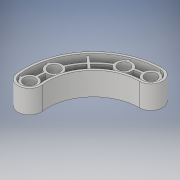
# Autodesk Inventor part: Curved_beam_6h-03
Saved by Autodesk Inventor 2019.3 (Build 233278000, 278)
## iProperties
Created: 2019-01-29
Part Number: Curved_beam_6h-03
Material: Generic
Document SubType Name: Modeling
Designer: Varga Daniel
Density: 1 g/cm^3
Appearance: Default
Inner_diameter: 40,000 mm
End_hole_dist: 37,500 mm
Author: Varga Daniel
Autodesk Inventor part; units mm, degrees
ref_plane "YZ Plane" through (0, 0, 0) normal (1, 0, 0) x (0, 1, 0)
ref_plane "XZ Plane" through (0, 0, 0) normal (0, 1, 0) x (-1, 0, 0)
ref_plane "XY Plane" through (0, 0, 0) normal (0, 0, 1) x (1, 0, 0)
derived "Base_part.ipt"
sketch "Sketch2" plane through (0, 0, 0) normal (0, 1, 0) x (-1, 0, 0)
  arc A0 (0, -20) -> (19.8431, 2.5) centre (0, 0) ccw
  arc A1 (0, -25) -> (24.8039, 3.125) centre (0, 0) ccw construction
  arc A2 (0, -30) -> (29.7647, 3.75) centre (0, 0) ccw
  line L0 (0, -20) -> (0, -30) construction
  line L1 (19.8431, 2.5) -> (29.7647, 3.75) construction
  arc A3 (0, -21) -> (20.8353, 2.625) centre (0, 0) ccw
  arc A4 (0, -29) -> (28.7725, 3.625) centre (0, 0) ccw
  circle A5 centre (0, -25) radius 3.5
  circle A6 centre (9.798, -23) radius 3.5
  arc A7 (0, -20) -> (0, -30) centre (0, -25) ccw
  arc A8 (0, -21) -> (0, -29) centre (0, -25) ccw
  arc A9 (29.7647, 3.75) -> (19.8431, 2.5) centre (24.8039, 3.125) ccw
  arc A10 (28.7725, 3.625) -> (20.8353, 2.625) centre (24.8039, 3.125) ccw
  circle A11 centre (24.8039, 3.125) radius 3.5
  circle A12 centre (24.0443, -6.8461) radius 3.5
  line L2 (0, 0) -> (22.5, -19.8431) construction
  arc A13 (24.6256, 6.6205) -> (24.488, 7.1125) centre (0, 0) ccw
  arc A14 (23.6421, 6.4265) -> (23.5058, 6.9085) centre (0, 0) ccw
  arc A15 (24.2694, -3.3534) -> (24.4973, -0.3615) centre (0, 0) ccw
  arc A16 (25.2502, -3.5604) -> (25.4982, -0.3055) centre (0, 0) ccw
  arc A17 (12.6551, -20.9785) -> (22.3958, -9.9336) centre (0, 0) ccw
  arc A18 (13.111, -21.8713) -> (23.3386, -10.2742) centre (0, 0) ccw
  arc A19 (-3.9161, -24.185) -> (-3.4209, -24.26) centre (0, 0) ccw
  arc A20 (3.4209, -24.26) -> (6.3607, -23.6599) centre (0, 0) ccw
  arc A21 (-3.9957, -25.185) -> (-3.4903, -25.26) centre (0, 0) ccw
  arc A22 (3.4903, -25.26) -> (6.6888, -24.6071) centre (0, 0) ccw
  line L3 (0, -25) -> (0, 0) construction
  line L4 (9.798, -23) -> (0, 0) construction
  line L5 (24.0443, -6.8461) -> (0, 0) construction
  line L6 (24.8039, 3.125) -> (0, 0) construction
  line L7 (7.768, -19.5105) -> (7.9803, -20.009)
  line L8 (10.6956, -26.3829) -> (10.9039, -26.872)
  line L9 (8.688, -19.1186) -> (8.9003, -19.6171)
  line L10 (11.6156, -25.991) -> (11.8239, -26.4801)
  line L11 (0.5, -20.994) -> (0.5, -21.5359)
  line L12 (0.5, -28.4641) -> (0.5, -28.9957)
  line L13 (-0.5, -28.9686) -> (-0.5, -28.4641)
  line L14 (-0.5, -21.5359) -> (-0.5, -21.0314)
  circle A23 centre (0, -25) radius 2.5
  circle A24 centre (9.798, -23) radius 2.5
  circle A25 centre (24.0443, -6.8461) radius 2.5
  circle A26 centre (24.8039, 3.125) radius 2.5
  line L15 (20.0546, -6.23) -> (20.5757, -6.3784)
  line L16 (27.2391, -8.2756) -> (27.7504, -8.4212)
  line L17 (20.3285, -5.2682) -> (20.8496, -5.4166)
  line L18 (27.513, -7.3138) -> (28.0242, -7.4594)
  line L19 (28.6789, 4.1172) -> (28.1784, 4.0541)
  line L20 (21.3045, 3.1881) -> (20.8039, 3.125)
  line L21 (20.8919, 2.1282) -> (21.4295, 2.1959)
  line L22 (28.3034, 3.0619) -> (28.8308, 3.1284)
  circle A27 centre (5, 5) radius 2.5 construction
  circle A28 centre (5, 5) radius 3.5 construction
  line L23 (15.4148, -14.2613) -> (18.0405, -16.5769)
  line L24 (18.7019, -15.8269) -> (16.0763, -13.5113)
  line L25 (18.7906, -17.2384) -> (21.416, -19.5538)
  line L26 (22.0775, -18.8038) -> (19.452, -16.4884)
  dimension "d84" = 7
  dimension "d85" = 7
  dimension "d86" = 7
  dimension "d87" = 7
  dimension "d0" = 20
  dimension "d5" = 1
  dimension "d14" = 10
  dimension "d15" = 4
  dimension "d21" = 10
  dimension "d34" = 1
  dimension "d35" = 0.5
  dimension "d37" = 1
  dimension "d38" = 1
  dimension "d45" = 5
  dimension "d51" = 1
  dimension "d53" = 1
  dimension "d77" = 4
  dimension "d78" = 4
  dimension "d79" = 5
  dimension "d80" = 7
  dimension "d81" = 5
  dimension "d82" = 5
  dimension "d83" = 5
  dimension "d88" = 1
  dimension "d89" = 37.5
  constraints: 54 end point, 51 point on circle, 21 centre point, 17 parallel, 12 coincident, 10 collinear, 8 concentric, 7 point on line, 3 midpoint, 2 vertical, 1 tangent, 74 other
  measures "d0" radius of A0
  measures "d14" distance of A1.start L4.start
  measures "d15" radius of A8
  measures "d21" distance of A9.centre L5.start
  measures "d34" radial gap between concentric circles of A20 A22
  measures "d35" radial gap between concentric circles of A1 A22
  measures "d37" distance between parallel lines of L14 L11
  measures "d38" distance between parallel lines of L7 L9
  measures "d45" diameter of A25
  measures "d51" distance between parallel lines of L17 L15
  measures "d53" distance between parallel lines of L20 L21
  measures "d79" diameter of A27
  measures "d80" diameter of A28
  measures "d81" diameter of A23
  measures "d82" diameter of A24
  measures "d83" diameter of A26
  measures "d88" distance between parallel lines of L24 L23
  measures "d89" distance of A1.end A1.start
extrude "Extrusion7" add sketch "Sketch2" along normal mid plane 8.4 contours A3 L11 A5 L14 A8 | A3 L9 A6 L7 | A5 | A19 A5 A21 A8 | A6 | A20 A6 A22 A5 | A3 L24 A17 L23 | L13 A5 L12 A4 A8 | A17 A12 A18 A6 | A3 L17 A12 L15 | A6 L10 A4 L8 | A12 | A18 L26 A4 L25 | A3 A10 L20 A11 L21 | A11 | A15 A11 A16 A12 | A12 L18 A4 L16 | A10 A13 A11 A14 | A11 L19 A10 A4 L22
extrude "Extrusion8" add sketch "Sketch2" along normal mid plane 1 contours A3 L7 A6 A20 A5 L11 | L14 A5 A19 A8 | A3 L23 A17 A6 L9 | A21 A5 L13 A8 | A3 L15 A12 A17 L24 | A6 L8 A4 L12 A5 A22 | A18 L25 A4 L10 A6 | A3 L21 A11 A15 A12 L17 | A12 L16 A4 L26 A18 | A10 A14 A11 L20 | A16 A11 L22 A4 L18 A12 | A10 L19 A11 A13
extrude "Extrusion9" add sketch "Sketch2" along normal mid plane 10 contours A0 A9 A2 A7
sketch "Sketch1" plane through (0, 0, 0) normal (0, 1, 0) x (-1, 0, 0)
  line L0 (5, 0) -> (25, 0) projected
  line L1 (30, 5) -> (30, 25) projected
  line L2 (25, 30) -> (5, 30) projected
  line L3 (0, 25) -> (0, 5) projected
  line L4 (5, 29) -> (25, 29) projected
  line L5 (29, 25) -> (29, 5) projected
  line L6 (25, 1) -> (5, 1) projected
  line L7 (1, 5) -> (1, 25) projected
  circle A0 centre (5, 5) radius 2.5 projected
  circle A1 centre (5, 5) radius 3.5 projected
  arc A2 (25, 0) -> (30, 5) centre (25, 5) ccw projected
  arc A3 (30, 25) -> (25, 30) centre (25, 25) ccw projected
  arc A4 (5, 30) -> (0, 25) centre (5, 25) ccw projected
  arc A5 (0, 5) -> (5, 0) centre (5, 5) ccw projected
  arc A6 (1, 5) -> (5, 1) centre (5, 5) ccw projected
  arc A7 (5, 29) -> (1, 25) centre (5, 25) ccw projected
  arc A8 (29, 25) -> (25, 29) centre (25, 25) ccw projected
  arc A9 (25, 1) -> (29, 5) centre (25, 5) ccw projected
  line L8 (49.1041, 15) -> (-27.081, 15) construction
  circle A10 centre (15, 5) radius 2.5
  circle A11 centre (15, 5) radius 3.5
  line L9 (31.1478, 10) -> (-2.4877, 10) construction
  line L10 (-2.8604, 5) -> (35.495, 5) construction
  line L11 (5, -2.5736) -> (5, 36.7522) construction
  line L12 (15, -1.4978) -> (15, 34.8784) construction
  line L13 (18.4641, 5.5) -> (21.5359, 5.5)
  line L14 (18.4641, 4.5) -> (21.5359, 4.5)
  line L15 (1.5359, 5.5) -> (1, 5.5) projected
  line L16 (1.5359, 4.5) -> (1.0314, 4.5) projected
  line L17 (28.9686, 4.5) -> (8.4641, 4.5) projected
  line L18 (29, 5.5) -> (8.4641, 5.5) projected
  line L19 (4.5, 1.5359) -> (4.5, 1.0314) projected
  line L20 (5.5, 1.5359) -> (5.5, 1) projected
  line L21 (29, 10.5) -> (1, 10.5) projected
  line L22 (29, 9.5) -> (1, 9.5) projected
  line L23 (4.5, 28.9686) -> (4.5, 10.5) projected
  line L24 (4.5, 9.5) -> (4.5, 8.4641) projected
  line L25 (5.5, 29) -> (5.5, 10.5) projected
  line L26 (5.5, 9.5) -> (5.5, 8.4641) projected
  point P0 (0, 0)
  point P1 (30, 30)
  point P2 (0, 30)
  constraints: 4 end point, 2 centre point, 1 other
equation "\"d5\" = Wall_thickness"
equation "\"d34\" = Inner_route_thickness"
equation "\"d35\" = 0.5 * d34"
equation "\"d37\" = Inner_route_thickness"
equation "\"d38\" = d37"
equation "\"d30\" = Inner_route_thickness"
equation "\"d31\" = 0.5 * d30"
equation "\"d32\" = Inner_route_thickness"
equation "\"d33\" = 0.5 * d32"
equation "\"d39\" = d40"
equation "\"d47\" = d37"
equation "\"Inner_diameter\" = 40"
equation "\"End_hole_dist\" = 37.5"
equation "\"Wall_thickness\" = 1"
equation "\"Inner_route_thickness\" = 1"
equation "\"d40\" = 5"
body "Solid2"
